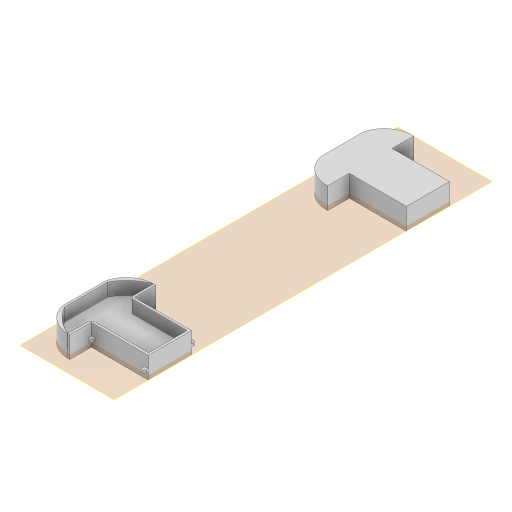
# Autodesk Inventor part: Part1
Saved by Autodesk Inventor 2024.3 (Build 283343000, 343)
## iProperties
Created: 2025-09-23
Part Number: Part1
Material: Generic
Document SubType Name: Modeling
Designer: danie
Density: 1 g/cm^3
Appearance: Default
Author: danie
Autodesk Inventor part; units mm, degrees
ref_plane "YZ Plane" through (0, 0, 0) normal (1, 0, 0) x (0, 1, 0)
ref_plane "XZ Plane" through (0, 0, 0) normal (0, 1, 0) x (-1, 0, 0)
ref_plane "XY Plane" through (0, 0, 0) normal (0, 0, 1) x (1, 0, 0)
sketch "Sketch1" plane through (0, 0, 0) normal (0, 1, 0) x (-1, 0, 0)
  line L0 (-60.8639, 0) -> (-200, 0)
  line L1 (-200, 0) -> (-200, -200)
  line L2 (-200, -200) -> (0, -200)
  line L3 (0, -200) -> (0, 0)
  line L4 (0, -200) -> (-200, -200)
  line L5 (-200, -200) -> (-200, -400)
  line L6 (-200, -400) -> (0, -400)
  line L7 (0, -400) -> (0, -200)
  line L8 (-60.8639, 0) -> (-67, 0)
  line L9 (0, -200) -> (0, -100)
  line L10 (0, -50) -> (0, -100)
  line L11 (0, -100) -> (0, -50)
  line L12 (0, -50) -> (0, -150)
  line L13 (0, -150) -> (-67, -150)
  line L14 (0, -50) -> (-67, -50)
  line L15 (-14.5617, -10.867) -> (0, 0)
  line L16 (-67, -150) -> (0, -200)
  arc A0 (0, -50) -> (-67, 0) centre (-63.932, -65.7788) ccw
  line L17 (0, -200) -> (15.754, -200)
  line L18 (15.754, -200) -> (0, -200)
  line L19 (0, -200) -> (0, -184.246)
  line L20 (0, -184.246) -> (-21.1104, -184.246)
  line L21 (-21.1104, -184.246) -> (-21.1104, -200)
  arc A1 (-67, -200) -> (0, -150) centre (-63.9339, -134.2186) ccw
  line L22 (-67, -50) -> (-200, -50)
  line L23 (-67, -150) -> (-200, -150)
  line L24 (-67, 0) -> (-67, -50)
  line L25 (-67, -150) -> (-67, -200)
  line L26 (-200, -800) -> (-200, -600)
  line L27 (0, -750) -> (0, -700)
  line L28 (0, -750) -> (0, -650)
  line L29 (0, -650) -> (-67, -650)
  line L30 (0, -750) -> (-67, -750)
  line L31 (-67, -650) -> (0, -600)
  arc A2 (-67, -800) -> (0, -750) centre (-63.932, -734.2212) ccw
  arc A3 (0, -650) -> (-67, -600) centre (-63.9339, -665.7814) ccw
  line L32 (-67, -750) -> (-200, -750)
  line L33 (-67, -650) -> (-200, -650)
  line L34 (-67, -800) -> (-67, -750)
  line L35 (-67, -650) -> (-67, -600)
  point P0 (-60.8677, -200)
  dimension "d0" = 200
  dimension "d1" = 200
  dimension "d2" = 200
  dimension "d3" = 200
  dimension "d4" = 67
  dimension "d5" = 100
  dimension "d6" = 50
  dimension "d7" = 100
  dimension "d8" = 15.754
  dimension "d9" = 15.754
  constraints: 72 end point, 14 symmetric about line, 13 perpendicular, 10 point on circle, 9 point on line, 4 centre point, 4 parallel, 2 collinear, 2 horizontal, 2 midpoint, 2 other
  measures "d0" distance of L2.end L1.end
  measures "d1" distance of L1.end L0.end
  measures "d2" distance of L6.end L5.end
  measures "d3" distance of L5.end L4.end
  measures "d4" distance of L3.end L8.end
  measures "d5" distance of L3.end L9.end
  measures "d6" distance of L10.start L9.end
  measures "d7" distance of L10.start L12.end
  measures "d8" distance of L2.end L17.end
  measures "d9" distance of L2.end L19.end
extrude "Extrusion1" add sketch "Sketch1" along normal blind 50 contours A0 L14 L24 L0 | L3 L13 L23 L1 L22 L14 | A1 L16 L13 | L16 A1 L2 L25 | L26 L33 L29 L28 L27 L30 L32 | L30 A2 L34 | L31 A3 L29 | L35 A3 L31
sketch "Sketch2" plane through (0, 50, 0) normal (0, 1, 0) x (1, 0, 0)
  line L0 (67, 50) -> (200, 50) projected
  line L1 (200, 50) -> (200, 150)
  line L2 (200, 150) -> (67, 150)
  line L3 (67, 150) -> (67, 199.2984)
  line L4 (67, 199.2984) -> (67, 200.0458)
  line L5 (0, 150) -> (0, 50) projected
  line L6 (0, 50) -> (0, 150)
  line L7 (67, 50) -> (200, 50)
  arc A0 (0, 50) -> (63.932, 0) centre (63.792, 65.694) ccw
  arc A1 (60.8677, 200) -> (0, 150) centre (63.9339, 134.2186) ccw projected
  arc A2 (67, 200.0458) -> (0, 150) centre (64.0367, 134.1412) ccw
  line L8 (107.1865, 50) -> (107.1865, 55)
  line L9 (107.1865, 55) -> (67, 55)
  line L10 (200, 55) -> (195, 55)
  line L11 (195, 150) -> (195, 145)
  line L12 (195, 145) -> (67, 145)
  line L13 (67, 145) -> (67, 55)
  line L14 (67, 55) -> (195, 55)
  line L15 (195, 55) -> (195, 145)
  line L16 (0, 102.5601) -> (5, 102.5601)
  line L17 (5, 102.5601) -> (5, 150)
  line L18 (67, 150) -> (67, 200) projected
  line L19 (67, 150) -> (62, 150)
  line L20 (62, 150) -> (5, 150)
  line L21 (62, 150) -> (62, 145)
  line L22 (62, 145) -> (72.629, 145)
  line L23 (67, 50) -> (62, 50)
  line L24 (62, 50) -> (62, 55)
  line L25 (62, 50) -> (5, 50)
  line L26 (5, 50) -> (5, 104.6986)
  line L27 (67, 55) -> (62, 55)
  line L28 (62, 50) -> (67, 55)
  line L29 (67, 145) -> (62, 150)
  line L30 (67, 200) -> (62.0007, 200.081)
  line L31 (62.0007, 200.081) -> (62, 150)
  arc A3 (62.0007, 200.081) -> (5, 150) centre (102.4081, 96.6117) ccw
  line L32 (62.0007, 50.0007) -> (62.0007, 0.0243)
  arc A4 (5, 50) -> (62.0007, 0.0243) centre (106.1149, 107.8339) ccw
  point P0 (0, 0)
  point P1 (62.0007, 50)
  dimension "d12" = 5
  dimension "d13" = 5
  dimension "d14" = 5
  dimension "d15" = 5
  dimension "d16" = 5
  dimension "d17" = 5
  dimension "d18" = 5
  constraints: 60 end point, 12 perpendicular, 10 point on circle, 9 point on line, 4 centre point, 4 horizontal, 2 collinear, 2 parallel, 2 vertical
  measures "d12" distance of L8.start L8.end
  measures "d13" distance of L10.start L10.end
  measures "d14" distance of L11.start L11.end
  measures "d15" distance of L16.start L16.end
  measures "d16" distance of L2.end L19.end
  measures "d17" distance of L0.start L23.end
  measures "d18" distance of L18.end L30.end
extrude "Extrusion2" cut sketch "Sketch2" against normal blind 30 contours L25 L26 L17 L20 L21 L22 L13 L27 L24 | L32 A4 L25 | L24 L27 L28 | L9 L13 L12 L15 L14 | L22 L21 L29 | L20 A3 L31
ref_plane "Work Plane1" through (0, 10, 0) normal (0, 1, 0) x (1, 0, 0)
sketch "Sketch3" plane through (0, 20, 0) normal (0, 1, 0) x (1, 0, 0)
  line L0 (67, 150) -> (200, 150) projected
  line L1 (200, 150) -> (200, 50) projected
  line L2 (200, 50) -> (67, 50) projected
  line L3 (67, 50) -> (67, 0) projected
  line L4 (67, 0) -> (60.8639, 0) projected
  arc A0 (0, 50) -> (60.8639, 0) centre (63.932, 65.7788) ccw projected
  line L5 (0, 50) -> (0, 150) projected
  arc A1 (60.8677, 200) -> (0, 150) centre (63.9339, 134.2186) ccw projected
  line L6 (60.8677, 200) -> (61.7939, 200) projected
  arc A2 (61.7939, 200) -> (5, 150) centre (102.4081, 96.6117) ccw projected
  line L7 (5, 150) -> (5, 50) projected
  arc A3 (5, 50) -> (62.0007, 0.0243) centre (106.1149, 107.8339) ccw projected
  line L8 (62.0007, 0.0243) -> (62.0007, 50) projected
  line L9 (62.0007, 50) -> (62, 50) projected
  line L10 (62, 50) -> (67, 55) projected
  line L11 (67, 55) -> (195, 55) projected
  line L12 (195, 55) -> (195, 145) projected
  line L13 (195, 145) -> (67, 145) projected
  line L14 (67, 145) -> (62, 150) projected
  line L15 (62, 150) -> (62.0007, 200) projected
  line L16 (61.7939, 200) -> (62.0007, 200) projected
  line L17 (67, 200) -> (67, 150) projected
  line L18 (62.0007, 200) -> (67, 200) projected
  arc A4 (0, 650) -> (67, 600) centre (63.9339, 665.7814) ccw projected
  line L19 (0, 650) -> (0, 750) projected
  arc A5 (67, 800) -> (0, 750) centre (63.932, 734.2212) ccw projected
  line L20 (67, 800) -> (67, 750) projected
  line L21 (67, 750) -> (200, 750) projected
  line L22 (200, 750) -> (200, 650) projected
  line L23 (200, 650) -> (67, 650) projected
  line L24 (67, 650) -> (67, 600) projected
  line L25 (67, 150) -> (200, 150) projected
  line L26 (200, 150) -> (200, 50) projected
  line L27 (200, 50) -> (67, 50) projected
  line L28 (67, 50) -> (67, 0) projected
  line L29 (67, 0) -> (60.8639, 0) projected
  arc A6 (0, 50) -> (60.8639, 0) centre (63.932, 65.7788) ccw projected
  line L30 (0, 50) -> (0, 150) projected
  arc A7 (60.8677, 200) -> (0, 150) centre (63.9339, 134.2186) ccw projected
  line L31 (60.8677, 200) -> (61.7939, 200) projected
  arc A8 (61.7939, 200) -> (5, 150) centre (102.4081, 96.6117) ccw projected
  line L32 (5, 150) -> (5, 50) projected
  arc A9 (5, 50) -> (62.0007, 0.0243) centre (106.1149, 107.8339) ccw projected
  line L33 (62.0007, 0.0243) -> (62.0007, 50) projected
  line L34 (62.0007, 50) -> (62, 50) projected
  line L35 (62, 50) -> (67, 55) projected
  line L36 (67, 55) -> (195, 55) projected
  line L37 (195, 55) -> (195, 145) projected
  line L38 (195, 145) -> (67, 145) projected
  line L39 (67, 145) -> (62, 150) projected
  line L40 (62, 150) -> (62.0007, 200) projected
  line L41 (61.7939, 200) -> (62.0007, 200) projected
  line L42 (67, 200) -> (67, 150) projected
  line L43 (62.0007, 200) -> (67, 200) projected
  arc A10 (0, 650) -> (67, 600) centre (63.9339, 665.7814) ccw projected
  line L44 (0, 650) -> (0, 750) projected
  arc A11 (67, 800) -> (0, 750) centre (63.932, 734.2212) ccw projected
  line L45 (67, 800) -> (67, 750) projected
  line L46 (67, 750) -> (200, 750) projected
  line L47 (200, 750) -> (200, 650) projected
  line L48 (200, 650) -> (67, 650) projected
  line L49 (67, 650) -> (67, 600) projected
  line L50 (67, 50) -> (200, 50) projected
  line L51 (67, 50) -> (77, 50)
  line L52 (77, 50) -> (77, 40)
  line L53 (77, 40) -> (67, 40)
  line L54 (67, 40) -> (67, 50)
  line L55 (200, 50) -> (190, 50)
  line L56 (190, 50) -> (190, 40)
  line L57 (190, 40) -> (200, 40)
  line L58 (200, 40) -> (200, 50)
  line L59 (200, 50) -> (200, 150) projected
  line L60 (200, 150) -> (190, 150)
  line L61 (190, 150) -> (190, 160)
  line L62 (190, 160) -> (200, 160)
  line L63 (200, 160) -> (200, 150)
  line L64 (67, 150) -> (77, 150)
  line L65 (77, 150) -> (77, 160)
  line L66 (77, 160) -> (67, 160)
  line L67 (67, 160) -> (67, 150)
  circle A12 centre (72, 45) radius 5
  circle A13 centre (195, 45) radius 5
  circle A14 centre (195, 155) radius 5
  circle A15 centre (72, 155) radius 5
  point P0 (0, 0)
  point P1 (67, 45)
  point P2 (77, 45)
  point P3 (190, 45)
  point P4 (200, 45)
  point P5 (190, 155)
  point P6 (200, 155)
  point P7 (77, 155)
  point P8 (67, 155)
  dimension "d21" = 10
  dimension "d22" = 10
  dimension "d23" = 10
  dimension "d24" = 10
  dimension "d25" = 10
  dimension "d26" = 10
  dimension "d27" = 10
  constraints: 32 end point, 8 parallel, 4 centre point, 4 horizontal, 4 perpendicular
  measures "d21" distance of L52.end L53.end
  measures "d22" distance of L51.end L52.end
  measures "d23" distance of L57.end L56.end
  measures "d24" distance of L56.end L55.end
  measures "d25" distance of L61.end L62.end
  measures "d26" distance of L60.end L61.end
  measures "d27" distance of L66.end L65.end
extrude "Extrusion3" add sketch "Sketch3" along normal mid plane 5.75 contours L0 A15 L65 | L61 A14 L0 | L0 L17 A15 | A15 | A14 L63 L0 | A14 | L58 A13 L2 | A13 L56 L2 | A13 | L52 A12 L2 | A12 L3 L2 | A12
body "Solid1"
